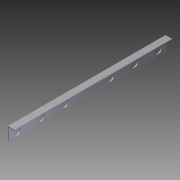
# Autodesk Inventor part: maipulator L frame front
Saved by Autodesk Inventor 2012 (Build 160160000, 160)
## iProperties
Created: 2013-09-01
Part Number: maipulator L frame front
Material: Default
Document SubType Name: Modeling
Designer: Bryce
Density: 1 g/cm^3
Author: Bryce
Autodesk Inventor part; units mm, degrees
ref_plane "YZ Plane" through (0, 0, 0) normal (1, 0, 0) x (0, 1, 0)
ref_plane "XZ Plane" through (0, 0, 0) normal (0, 1, 0) x (-1, 0, 0)
ref_plane "XY Plane" through (0, 0, 0) normal (0, 0, 1) x (1, 0, 0)
sketch "Sketch1" plane through (0, 0, 0) normal (0, 0, 1) x (1, 0, 0)
  line L0 (0, 0) -> (25.4, 0)
  line L1 (25.4, 0) -> (25.4, 3.175)
  line L2 (3.175, 50.8) -> (0, 50.8)
  line L3 (0, 50.8) -> (0, 0)
  line L4 (3.175, 50.8) -> (3.175, 3.175)
  line L5 (3.175, 3.175) -> (25.4, 3.175)
  dimension "d0" = 50.8
  dimension "d1" = 25.4
  dimension "d2" = 3.175
  dimension "d3" = 3.175
  constraints: 12 end point, 2 parallel, 1 horizontal, 1 perpendicular
  measures "d0" distance of L2.end L0.start
  measures "d1" distance of L0.start L0.end
  measures "d2" distance between parallel lines of L4 L3
  measures "d3" distance between parallel lines of L0 L5
extrude "Extrusion1" add sketch "Sketch1" along normal blind 609.6
sketch "Sketch2" plane through (0, 0, 0) normal (-1, 0, 0) x (0, 0, 1)
  line L0 (609.6, 0) -> (609.6, 50.8) projected
  line L1 (0, 50.8) -> (609.6, 50.8) projected
  line L2 (0, 50.8) -> (0, 0) projected
  circle A0 centre (577.85, 31.75) radius 14.2875
  circle A1 centre (393.7, 31.75) radius 14.2875
  circle A2 centre (215.9, 31.75) radius 14.2875
  circle A3 centre (31.75, 31.75) radius 14.2875
  circle A4 centre (485.775, 31.75) radius 14.2875
  circle A5 centre (123.825, 31.75) radius 14.2875
  dimension "d6" = 28.575
  dimension "d7" = 31.75
  dimension "d8" = 19.05
  dimension "d9" = 28.575
  dimension "d10" = 177.8
  dimension "d11" = 31.75
  dimension "d15" = 184.15
  dimension "d16" = 92.075
  dimension "d17" = 92.075
  dimension "d18" = 609.6
  constraints: 6 centre point, 5 horizontal alignment, 4 equal radius
  measures "d6" diameter of A0
  measures "d7" distance from line of L0 A0.centre
  measures "d8" distance from line of L1 A0.centre
  measures "d9" diameter of A1
  measures "d10" distance of A2.centre A1.centre
  measures "d11" distance from line of L2 A3.centre
  measures "d15" distance of A1.centre A0.centre
  measures "d16" distance of A4.centre A0.centre
  measures "d17" distance of A5.centre A2.centre
  measures "d18" distance between parallel lines of L2 L0
extrude "Extrusion2" cut sketch "Sketch2" against normal through all
equation "\"d2\" = d3"
equation "\"d11\" = d7"
equation "\"d15\" = 0.5 * d18 - 0.5 * d10 - d7"
equation "\"d16\" = 0.5 * d15"
equation "\"d17\" = d16"
body "Solid1"
